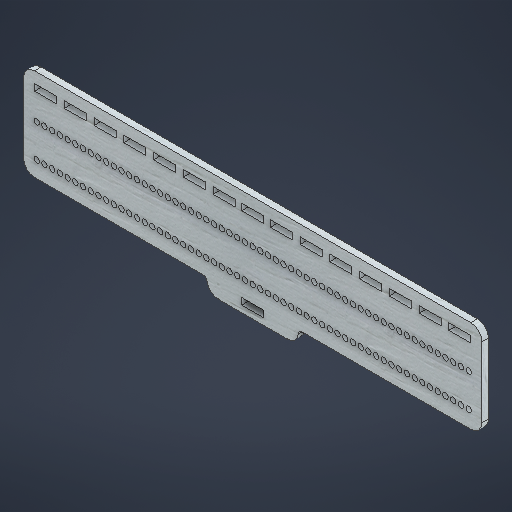
# Autodesk Inventor part: side_frame_test
Saved by Autodesk Inventor 2025.3 (Build 293356030, 356C)
## iProperties
Created: 2025-09-04
Part Number: side_frame_test
Material: 木材 (楓木)
Document SubType Name: Modeling
Designer: 陳泓任
Density: 0.67 g/cm^3
Appearance: 木材 - 白色刷漆
Author: 陳泓任
Autodesk Inventor part; units mm, degrees
ref_plane "YZ Plane" through (0, 0, 0) normal (1, 0, 0) x (0, 1, 0)
ref_plane "XZ Plane" through (0, 0, 0) normal (0, 1, 0) x (-1, 0, 0)
ref_plane "XY Plane" through (0, 0, 0) normal (0, 0, 1) x (1, 0, 0)
sketch "草圖1" plane through (0, 0, 0) normal (0, 0, 1) x (1, 0, 0)
  arc A0 (99, -14.8985) -> (104, -9.8985) centre (99, -9.8985) ccw
  arc A1 (-104, -9.8985) -> (-99, -14.8985) centre (-99, -9.8985) ccw
  circle A2 centre (0, 7.5) radius 1.25
  circle A3 centre (0, -7.5) radius 1.25
  line L0 (-99, -14.8985) -> (-22.615, -14.8985)
  arc A4 (15.6624, -21.0852) -> (20.6286, -16.6661) centre (15.6624, -16.0852) ccw
  arc A5 (22.615, -14.8985) -> (20.6286, -16.6661) centre (22.615, -16.8985) ccw
  line L1 (-5, -18.0852) -> (-5, -15.0852)
  line L2 (-5, -15.0852) -> (5, -15.0852)
  line L3 (5, -15.0852) -> (5, -18.0852)
  line L4 (5, -18.0852) -> (-5, -18.0852)
  arc A6 (-20.6286, -16.6661) -> (-22.615, -14.8985) centre (-22.615, -16.8985) ccw
  arc A7 (-20.6286, -16.6661) -> (-15.6624, -21.0852) centre (-15.6624, -16.0852) ccw
  line L5 (-15.6624, -21.0852) -> (15.6624, -21.0852)
  line L6 (22.615, -14.8985) -> (99, -14.8985)
  line L7 (0, -35.3826) -> (0, 51.5191) construction
  line L8 (-104.9871, 0) -> (119.3176, 0) construction
  line L9 (0, 7.5) -> (0, -7.5)
  circle A8 centre (3.5, 7.5) radius 1.25
  circle A9 centre (3.5, -7.5) radius 1.25
  circle A10 centre (-3.5, 7.5) radius 1.25
  circle A11 centre (-3.5, -7.5) radius 1.25
  circle A12 centre (7, 7.5) radius 1.25
  circle A13 centre (7, -7.5) radius 1.25
  circle A14 centre (-7, 7.5) radius 1.25
  circle A15 centre (-7, -7.5) radius 1.25
  circle A16 centre (10.5, 7.5) radius 1.25
  circle A17 centre (10.5, -7.5) radius 1.25
  circle A18 centre (-10.5, 7.5) radius 1.25
  circle A19 centre (-10.5, -7.5) radius 1.25
  circle A20 centre (14, 7.5) radius 1.25
  circle A21 centre (14, -7.5) radius 1.25
  circle A22 centre (-14, 7.5) radius 1.25
  circle A23 centre (-14, -7.5) radius 1.25
  circle A24 centre (17.5, 7.5) radius 1.25
  circle A25 centre (17.5, -7.5) radius 1.25
  circle A26 centre (-17.5, 7.5) radius 1.25
  circle A27 centre (-17.5, -7.5) radius 1.25
  circle A28 centre (21, 7.5) radius 1.25
  circle A29 centre (21, -7.5) radius 1.25
  circle A30 centre (-21, 7.5) radius 1.25
  circle A31 centre (-21, -7.5) radius 1.25
  circle A32 centre (24.5, 7.5) radius 1.25
  circle A33 centre (24.5, -7.5) radius 1.25
  circle A34 centre (-24.5, 7.5) radius 1.25
  circle A35 centre (-24.5, -7.5) radius 1.25
  circle A36 centre (28, 7.5) radius 1.25
  circle A37 centre (28, -7.5) radius 1.25
  circle A38 centre (-28, 7.5) radius 1.25
  circle A39 centre (-28, -7.5) radius 1.25
  circle A40 centre (31.5, 7.5) radius 1.25
  circle A41 centre (31.5, -7.5) radius 1.25
  circle A42 centre (-31.5, 7.5) radius 1.25
  circle A43 centre (-31.5, -7.5) radius 1.25
  circle A44 centre (35, 7.5) radius 1.25
  circle A45 centre (35, -7.5) radius 1.25
  circle A46 centre (-35, 7.5) radius 1.25
  circle A47 centre (-35, -7.5) radius 1.25
  circle A48 centre (38.5, 7.5) radius 1.25
  circle A49 centre (38.5, -7.5) radius 1.25
  circle A50 centre (-38.5, 7.5) radius 1.25
  circle A51 centre (-38.5, -7.5) radius 1.25
  circle A52 centre (42, 7.5) radius 1.25
  circle A53 centre (42, -7.5) radius 1.25
  circle A54 centre (-42, 7.5) radius 1.25
  circle A55 centre (-42, -7.5) radius 1.25
  circle A56 centre (45.5, 7.5) radius 1.25
  circle A57 centre (45.5, -7.5) radius 1.25
  circle A58 centre (-45.5, 7.5) radius 1.25
  circle A59 centre (-45.5, -7.5) radius 1.25
  circle A60 centre (49, 7.5) radius 1.25
  circle A61 centre (49, -7.5) radius 1.25
  circle A62 centre (-49, 7.5) radius 1.25
  circle A63 centre (-49, -7.5) radius 1.25
  circle A64 centre (52.5, 7.5) radius 1.25
  circle A65 centre (52.5, -7.5) radius 1.25
  circle A66 centre (-52.5, 7.5) radius 1.25
  circle A67 centre (-52.5, -7.5) radius 1.25
  circle A68 centre (56, 7.5) radius 1.25
  circle A69 centre (56, -7.5) radius 1.25
  circle A70 centre (-56, 7.5) radius 1.25
  circle A71 centre (-56, -7.5) radius 1.25
  circle A72 centre (59.5, 7.5) radius 1.25
  circle A73 centre (59.5, -7.5) radius 1.25
  circle A74 centre (-59.5, 7.5) radius 1.25
  circle A75 centre (-59.5, -7.5) radius 1.25
  circle A76 centre (63, 7.5) radius 1.25
  circle A77 centre (63, -7.5) radius 1.25
  circle A78 centre (-63, 7.5) radius 1.25
  circle A79 centre (-63, -7.5) radius 1.25
  circle A80 centre (66.5, 7.5) radius 1.25
  circle A81 centre (66.5, -7.5) radius 1.25
  circle A82 centre (-66.5, 7.5) radius 1.25
  circle A83 centre (-66.5, -7.5) radius 1.25
  circle A84 centre (70, 7.5) radius 1.25
  circle A85 centre (70, -7.5) radius 1.25
  circle A86 centre (-70, 7.5) radius 1.25
  circle A87 centre (-70, -7.5) radius 1.25
  circle A88 centre (73.5, 7.5) radius 1.25
  circle A89 centre (73.5, -7.5) radius 1.25
  circle A90 centre (-73.5, 7.5) radius 1.25
  circle A91 centre (-73.5, -7.5) radius 1.25
  circle A92 centre (77, 7.5) radius 1.25
  circle A93 centre (77, -7.5) radius 1.25
  circle A94 centre (-77, 7.5) radius 1.25
  circle A95 centre (-77, -7.5) radius 1.25
  circle A96 centre (80.5, 7.5) radius 1.25
  circle A97 centre (80.5, -7.5) radius 1.25
  circle A98 centre (-80.5, 7.5) radius 1.25
  circle A99 centre (-80.5, -7.5) radius 1.25
  circle A100 centre (84, 7.5) radius 1.25
  circle A101 centre (84, -7.5) radius 1.25
  circle A102 centre (-84, 7.5) radius 1.25
  circle A103 centre (-84, -7.5) radius 1.25
  circle A104 centre (87.5, 7.5) radius 1.25
  circle A105 centre (87.5, -7.5) radius 1.25
  circle A106 centre (-87.5, 7.5) radius 1.25
  circle A107 centre (-87.5, -7.5) radius 1.25
  circle A108 centre (91, 7.5) radius 1.25
  circle A109 centre (91, -7.5) radius 1.25
  circle A110 centre (-91, 7.5) radius 1.25
  circle A111 centre (-91, -7.5) radius 1.25
  circle A112 centre (94.5, 7.5) radius 1.25
  circle A113 centre (94.5, -7.5) radius 1.25
  circle A114 centre (-94.5, 7.5) radius 1.25
  circle A115 centre (-94.5, -7.5) radius 1.25
  circle A116 centre (98, 7.5) radius 1.25
  circle A117 centre (98, -7.5) radius 1.25
  circle A118 centre (-98, 7.5) radius 1.25
  circle A119 centre (-98, -7.5) radius 1.25
  line L10 (-99, 27) -> (99, 27)
  line L11 (-104, -9.8985) -> (-104, 22)
  line L12 (104, 22) -> (104, -9.8985)
  arc A120 (-99, 27) -> (-104, 22) centre (-99, 22) ccw
  arc A121 (104, 22) -> (99, 27) centre (99, 22) ccw
  line L13 (-99, 19) -> (-99, 22)
  line L14 (-99, 22) -> (-89, 22)
  line L15 (-89, 22) -> (-89, 19)
  line L16 (-89, 19) -> (-99, 19)
  line L17 (-5, 19) -> (5, 19)
  line L18 (5, 19) -> (5, 22)
  line L19 (5, 22) -> (-5, 22)
  line L20 (-5, 22) -> (-5, 19)
  line L21 (-5, 19) -> (5, 22) construction
  line L22 (5, 19) -> (-5, 22) construction
  line L23 (99, 22) -> (89, 22)
  line L24 (89, 22) -> (89, 19)
  line L25 (89, 19) -> (99, 19)
  line L26 (99, 19) -> (99, 22)
  line L27 (-85.5, 22) -> (-75.5, 22)
  line L28 (-85.5, 19) -> (-85.5, 22)
  line L29 (-75.5, 19) -> (-85.5, 19)
  line L30 (-75.5, 22) -> (-75.5, 19)
  line L31 (-72, 22) -> (-62, 22)
  line L32 (-72, 19) -> (-72, 22)
  line L33 (-62, 19) -> (-72, 19)
  line L34 (-62, 22) -> (-62, 19)
  line L35 (-58.5, 22) -> (-48.5, 22)
  line L36 (-58.5, 19) -> (-58.5, 22)
  line L37 (-48.5, 19) -> (-58.5, 19)
  line L38 (-48.5, 22) -> (-48.5, 19)
  line L39 (-45, 22) -> (-35, 22)
  line L40 (-45, 19) -> (-45, 22)
  line L41 (-35, 19) -> (-45, 19)
  line L42 (-35, 22) -> (-35, 19)
  line L43 (-31.5, 22) -> (-21.5, 22)
  line L44 (-31.5, 19) -> (-31.5, 22)
  line L45 (-21.5, 19) -> (-31.5, 19)
  line L46 (-21.5, 22) -> (-21.5, 19)
  line L47 (-18, 22) -> (-8, 22)
  line L48 (-18, 19) -> (-18, 22)
  line L49 (-8, 19) -> (-18, 19)
  line L50 (-8, 22) -> (-8, 19)
  line L51 (85.5, 22) -> (75.5, 22)
  line L52 (85.5, 19) -> (85.5, 22)
  line L53 (75.5, 19) -> (85.5, 19)
  line L54 (75.5, 22) -> (75.5, 19)
  line L55 (72, 22) -> (62, 22)
  line L56 (72, 19) -> (72, 22)
  line L57 (62, 19) -> (72, 19)
  line L58 (62, 22) -> (62, 19)
  line L59 (58.5, 22) -> (48.5, 22)
  line L60 (58.5, 19) -> (58.5, 22)
  line L61 (48.5, 19) -> (58.5, 19)
  line L62 (48.5, 22) -> (48.5, 19)
  line L63 (45, 22) -> (35, 22)
  line L64 (45, 19) -> (45, 22)
  line L65 (35, 19) -> (45, 19)
  line L66 (35, 22) -> (35, 19)
  line L67 (31.5, 22) -> (21.5, 22)
  line L68 (31.5, 19) -> (31.5, 22)
  line L69 (21.5, 19) -> (31.5, 19)
  line L70 (21.5, 22) -> (21.5, 19)
  line L71 (18, 22) -> (8, 22)
  line L72 (18, 19) -> (18, 22)
  line L73 (8, 19) -> (18, 19)
  line L74 (8, 22) -> (8, 19)
  point P0 (0, 0)
  point P1 (0, -15.0852)
  point P2 (0, 20.5)
  dimension "d0" = 10
  dimension "d1" = 3
  dimension "d2" = 3
  dimension "d4" = 2.5
  dimension "d12" = 2
  dimension "d16" = 15
  dimension "d29" = 45.23
  dimension "d30" = 31.3249
  dimension "d92" = 3.5
  dimension "d97" = 7.3985
  dimension "d98" = 5
  dimension "d100" = 208
  dimension "d101" = 19.5
  dimension "d102" = 5
  dimension "d107" = 10
  dimension "d108" = 3
  dimension "d118" = 13.5
  constraints: 150 end point, 122 centre point, 35 symmetric about line, 32 point on line, 16 point on circle, 14 tangent, 8 horizontal, 7 perpendicular, 6 equal radius, 3 collinear, 3 vertical, 2 equal length, 2 midpoint, 2 parallel, 281 other
  measures "d0" distance of L3.end L1.start
  measures "d1" distance of L1.start L1.end
  measures "d2" distance between parallel lines of L5 L4
  measures "d4" diameter of A2
  measures "d12" radius of A6
  measures "d16" distance of L9.end L9.start
  measures "d29" distance of A5.centre A6.centre
  measures "d30" distance of L5.start L5.end
  measures "d92" distance of L9.start A8.centre
  measures "d97" distance from line of L6 A109.centre
  measures "d98" radius of A1
  measures "d100" diameter of L11 L7
  measures "d101" distance from line of L10 A104.centre
  measures "d102" radius of A120
  measures "d107" distance of L15.end L16.end
  measures "d108" distance of L16.end L14.start
  measures "d118" distance of L14.start L27.start
extrude "擠出1" add sketch "草圖1" along normal mid plane 3
sketch "草圖3" plane through (0, 0, 1.5) normal (0, 0, 1) x (1, 0, 0)
  line L0 (0, 52.3829) -> (0, -39.0235)
  line L1 (-112.5881, 0) -> (123.4866, 0)
  point P0 (0, 0)
  constraints: 4 end point, 2 point on line, 1 horizontal, 1 vertical
